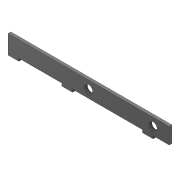
# Autodesk Inventor part: Divisória-30cm c rolamento
Saved by Autodesk Inventor 2020 (Build 240168000, 168)
## iProperties
Created: 2021-09-21
Part Number: Divisória-30cm c rolamento
Material: Generic
Document SubType Name: Modeling
Designer: pablo
Density: 1 g/cm^3
Appearance: Smooth - Black
Author: pablo
Autodesk Inventor part; units mm, degrees
ref_plane "YZ Plane" through (0, 0, 0) normal (1, 0, 0) x (0, 1, 0)
ref_plane "XZ Plane" through (0, 0, 0) normal (0, 1, 0) x (-1, 0, 0)
ref_plane "XY Plane" through (0, 0, 0) normal (0, 0, 1) x (1, 0, 0)
sketch "Sketch1" plane through (0, 0, 0) normal (0, 0, 1) x (1, 0, 0)
  line L0 (-150, 15) -> (150, 15)
  line L1 (150, 15) -> (150, -15)
  line L2 (150, -15) -> (-150, -15)
  line L3 (-150, -15) -> (-150, 15)
  line L4 (-150, 15) -> (150, -15) construction
  line L5 (150, 15) -> (-150, -15) construction
  point P0 (0, 0)
  dimension "d0" = 300
  dimension "d1" = 30
  constraints: 12 end point, 2 midpoint, 2 parallel, 1 horizontal, 1 perpendicular
  measures "d0" distance of L1.end L2.end
  measures "d1" distance of L0.end L1.end
extrude "Base" add sketch "Sketch1" along normal blind 5
sketch "Sketch2" plane through (0, 0, 5) normal (0, 0, 1) x (1, 0, 0)
  line L0 (-150, -15) -> (150, -15) projected
  line L1 (-150, -15) -> (-130, -15)
  line L2 (-130, -15) -> (-130, -20)
  line L3 (-130, -20) -> (-150, -20)
  line L4 (-150, -20) -> (-150, -15)
  line L5 (-100, -15) -> (-80, -15)
  line L6 (-80, -15) -> (-80, -20)
  line L7 (-80, -20) -> (-100, -20)
  line L8 (-100, -20) -> (-100, -15)
  line L9 (-50, -15) -> (-30, -15)
  line L10 (-30, -15) -> (-30, -20)
  line L11 (-30, -20) -> (-50, -20)
  line L12 (-50, -20) -> (-50, -15)
  line L13 (0, -15) -> (20, -15)
  line L14 (20, -15) -> (20, -20)
  line L15 (20, -20) -> (0, -20)
  line L16 (0, -20) -> (0, -15)
  line L17 (50, -15) -> (70, -15)
  line L18 (70, -15) -> (70, -20)
  line L19 (70, -20) -> (50, -20)
  line L20 (50, -20) -> (50, -15)
  line L21 (100, -15) -> (120, -15)
  line L22 (120, -15) -> (120, -20)
  line L23 (120, -20) -> (100, -20)
  line L24 (100, -20) -> (100, -15)
  point P0 (0, 0)
  point P1 (20, -15)
  point P2 (0, -15)
  point P3 (-30, -15)
  point P4 (-50, -15)
  point P5 (-130, -15)
  point P6 (70, -15)
  point P7 (50, -15)
  point P8 (-80, -15)
  point P9 (-100, -15)
  point P10 (120, -15)
  point P11 (100, -15)
  dimension "d4" = 20
  dimension "d5" = 5
  dimension "d8" = 50
  constraints: 48 end point, 2 horizontal, 2 parallel, 1 perpendicular, 40 other
  measures "d4" distance of L2.end L3.end
  measures "d5" distance of L1.end L2.end
  measures "d8" distance of L2.end L6.end
extrude "Encaixe" add sketch "Sketch2" against normal blind 5 contours L0 L22 L23 L24 | L0 L10 L11 L12 | L0 L2 L3 L4
sketch "Sketch3" plane through (0, 0, 5) normal (0, 0, 1) x (1, 0, 0)
  circle A0 centre (120, 0) radius 7.5
  circle A1 centre (0, 0) radius 7.5
  line L0 (150, -15) -> (150, 15) projected
  dimension "d16" = 15
  dimension "d17" = 15
  dimension "d20" = 30
  constraints: 2 centre point, 1 coincident
  measures "d16" diameter of A0
  measures "d17" diameter of A1
  measures "d20" distance from line of L0 A0.centre
extrude "Extrusion3" cut sketch "Sketch3" against normal blind 10
body "Solid1"
